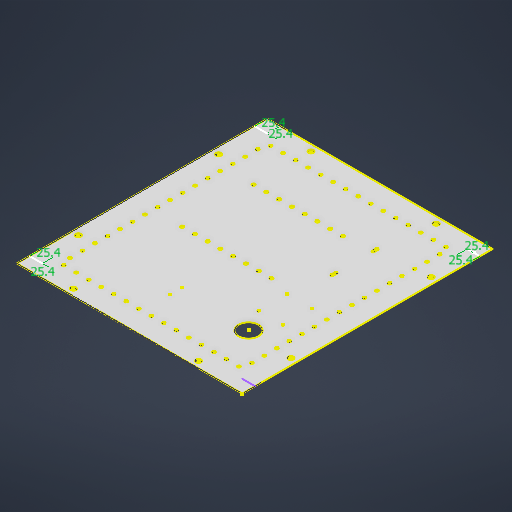
# Autodesk Inventor part: placa_dany
Saved by Autodesk Inventor 2026 (Build 300175050, 175E)
## iProperties
Created: 2025-11-18
Part Number: placa_dany
Material: Genérico
Document SubType Name: Modeling
Designer: sebas
Density: 1 g/cm^3
Appearance: Valor por defecto
Author: sebas
Autodesk Inventor part; units mm, degrees
ref_plane "YZ Plane" through (0, 0, 0) normal (1, 0, 0) x (0, 1, 0)
ref_plane "XZ Plane" through (0, 0, 0) normal (0, 1, 0) x (-1, 0, 0)
ref_plane "XY Plane" through (0, 0, 0) normal (0, 0, 1) x (1, 0, 0)
sketch "Boceto1" plane through (0, 0, 0) normal (0, 1, 0) x (-1, 0, 0)
  line L0 (0, 0) -> (450, 0)
  line L1 (450, 0) -> (450, -500)
  line L2 (450, -500) -> (0, -500)
  line L3 (0, -500) -> (0, 0)
  dimension "d0" = 450
  dimension "d1" = 500
  constraints: 8 end point, 2 parallel, 1 horizontal, 1 perpendicular
  measures "d0" distance of L1.end L2.end
  measures "d1" distance of L0.end L1.end
extrude "Extrusión1" add sketch "Boceto1" along normal blind 1.8
sketch "Boceto2" plane through (0, 1.8, 0) normal (0, 1, 0) x (1, 0, 0)
  line L0 (-450, 500) -> (-450, 0) projected
  line L1 (-450, 0) -> (0, 0) projected
  line L2 (-450, 0) -> (-450, 359)
  line L3 (0, 500) -> (-450, 500) projected
  line L4 (0, 0) -> (0, 500) projected
  line L5 (-348.5135, 228.3629) -> (-148.5135, 228.3629) construction
  circle A0 centre (-348.5135, 228.3629) radius 3
  circle A1 centre (-323.0135, 228.3629) radius 3
  circle A2 centre (-297.5135, 228.3629) radius 3
  circle A3 centre (-272.0135, 228.3629) radius 3
  circle A4 centre (-246.5135, 228.3629) radius 3
  circle A5 centre (-221.0135, 228.3629) radius 3
  circle A6 centre (-195.5135, 228.3629) radius 3
  circle A7 centre (-170.0135, 228.3629) radius 3
  line L6 (-345.4268, 372.6129) -> (-145.4268, 372.6129) construction
  circle A8 centre (-350, 372.6129) radius 3
  circle A9 centre (-324.5, 372.6129) radius 3
  circle A10 centre (-299, 372.6129) radius 3
  circle A11 centre (-273.5, 372.6129) radius 3
  circle A12 centre (-248, 372.6129) radius 3
  circle A13 centre (-222.5, 372.6129) radius 3
  circle A14 centre (-197, 372.6129) radius 3
  circle A15 centre (-171.5, 372.6129) radius 3
  line L7 (-400, 43.4) -> (-43, 43.4) construction
  circle A16 centre (-400, 43.4) radius 2.75
  circle A17 centre (-375, 43.4) radius 2.75
  circle A18 centre (-350, 43.4) radius 2.75
  circle A19 centre (-325, 43.4) radius 2.75
  circle A20 centre (-300, 43.4) radius 2.75
  circle A21 centre (-275, 43.4) radius 2.75
  circle A22 centre (-250, 43.4) radius 2.75
  circle A23 centre (-225, 43.4) radius 2.75
  circle A24 centre (-200, 43.4) radius 2.75
  circle A25 centre (-175, 43.4) radius 2.75
  circle A26 centre (-150, 43.4) radius 2.75
  circle A27 centre (-125, 43.4) radius 2.75
  circle A28 centre (-100, 43.4) radius 2.75
  circle A29 centre (-75, 43.4) radius 2.75
  circle A30 centre (-50, 43.4) radius 2.75
  line L8 (-406.6, 44.1958) -> (-406.6, 451.7958) construction
  circle A31 centre (-406.6, 62.5) radius 2.75
  circle A32 centre (-406.6, 87.5) radius 2.75
  circle A33 centre (-406.6, 112.5) radius 2.75
  circle A34 centre (-406.6, 137.5) radius 2.75
  circle A35 centre (-406.6, 162.5) radius 2.75
  circle A36 centre (-406.6, 187.5) radius 2.75
  circle A37 centre (-406.6, 212.5) radius 2.75
  circle A38 centre (-406.6, 237.5) radius 2.75
  circle A39 centre (-406.6, 262.5) radius 2.75
  circle A40 centre (-406.6, 287.5) radius 2.75
  circle A41 centre (-406.6, 312.5) radius 2.75
  circle A42 centre (-406.6, 337.5) radius 2.75
  circle A43 centre (-406.6, 362.5) radius 2.75
  circle A44 centre (-406.6, 387.5) radius 2.75
  circle A45 centre (-406.6, 412.5) radius 2.75
  circle A46 centre (-406.6, 437.5) radius 2.75
  line L9 (-406.6, 456.6) -> (-38, 456.6) construction
  circle A47 centre (-43.4, 62.5) radius 2.75
  circle A48 centre (-43.4, 87.5) radius 2.75
  circle A49 centre (-43.4, 112.5) radius 2.75
  circle A50 centre (-43.4, 137.5) radius 2.75
  circle A51 centre (-43.4, 162.5) radius 2.75
  circle A52 centre (-43.4, 187.5) radius 2.75
  circle A53 centre (-43.4, 212.5) radius 2.75
  circle A54 centre (-43.4, 237.5) radius 2.75
  circle A55 centre (-43.4, 262.5) radius 2.75
  circle A56 centre (-43.4, 287.5) radius 2.75
  circle A57 centre (-43.4, 312.5) radius 2.75
  circle A58 centre (-43.4, 337.5) radius 2.75
  circle A59 centre (-43.4, 362.5) radius 2.75
  circle A60 centre (-43.4, 387.5) radius 2.75
  circle A61 centre (-43.4, 412.5) radius 2.75
  circle A62 centre (-43.4, 437.5) radius 2.75
  line L10 (-400, 456.6) -> (-43, 456.6) construction
  circle A63 centre (-400, 456.6) radius 2.75
  circle A64 centre (-375, 456.6) radius 2.75
  circle A65 centre (-350, 456.6) radius 2.75
  circle A66 centre (-325, 456.6) radius 2.75
  circle A67 centre (-300, 456.6) radius 2.75
  circle A68 centre (-275, 456.6) radius 2.75
  circle A69 centre (-250, 456.6) radius 2.75
  circle A70 centre (-225, 456.6) radius 2.75
  circle A71 centre (-200, 456.6) radius 2.75
  circle A72 centre (-175, 456.6) radius 2.75
  circle A73 centre (-150, 456.6) radius 2.75
  circle A74 centre (-125, 456.6) radius 2.75
  circle A75 centre (-100, 456.6) radius 2.75
  circle A76 centre (-75, 456.6) radius 2.75
  circle A77 centre (-50, 456.6) radius 2.75
  arc A78 (-112.7335, 384.14) -> (-117.1835, 384.14) centre (-114.9585, 384.14) ccw
  arc A79 (-117.1835, 294.14) -> (-112.7335, 294.14) centre (-114.9585, 294.14) ccw
  arc A80 (-117.1835, 376.14) -> (-112.7335, 376.14) centre (-114.9585, 376.14) ccw
  arc A81 (-112.7335, 302.14) -> (-117.1835, 302.14) centre (-114.9585, 302.14) ccw
  line L11 (-117.1835, 384.14) -> (-117.1835, 376.14)
  line L12 (-112.7335, 376.14) -> (-112.7335, 384.14)
  line L13 (-117.1835, 302.14) -> (-117.1835, 294.14)
  line L14 (-112.7335, 294.14) -> (-112.7335, 302.14)
  circle A82 centre (-126.3146, 216.4498) radius 1.5
  circle A83 centre (-77.1746, 216.4498) radius 1.5
  circle A84 centre (-126.3146, 158.7698) radius 1.5
  circle A85 centre (-77.1746, 158.7698) radius 1.5
  circle A86 centre (-243.1932, 122.0864) radius 1
  circle A87 centre (-243.1932, 99.0264) radius 1
  circle A88 centre (-102.75, 115.25) radius 20
  circle A89 centre (-350, 487.3) radius 5
  circle A90 centre (-100, 487.3) radius 5
  circle A91 centre (-350, 12.7) radius 5
  circle A92 centre (-100, 12.7) radius 5
  circle A93 centre (-437.3, 390) radius 5
  circle A94 centre (-437.3, 110) radius 5
  circle A95 centre (-12.7, 390) radius 5
  circle A96 centre (-12.7, 110) radius 5
  point P0 (-43.4, 451.7958)
  point P1 (-406.6, 455.8042)
  dimension "d16" = 25.5
  dimension "d30" = 25.5
  dimension "d41" = 5.5
  dimension "d44" = 25
  dimension "d50" = 5.5
  dimension "d54" = 25
  dimension "d65" = 144.25
  dimension "d85" = 4.45
  dimension "d89" = 4.45
  dimension "d92" = 4.45
  dimension "d93" = 90
  dimension "d94" = 4.45
  dimension "d95" = 8
  dimension "d96" = 8
  dimension "d97" = 3
  dimension "d98" = 3
  dimension "d99" = 49.14
  dimension "d100" = 3
  dimension "d101" = 57.68
  dimension "d102" = 3
  dimension "d103" = 2
  dimension "d104" = 2
  dimension "d105" = 23.06
  dimension "d106" = 40
  dimension "d113" = 10
  dimension "d114" = 10
  dimension "d115" = 10
  dimension "d116" = 10
  dimension "d117" = 10
  dimension "d118" = 10
  dimension "d119" = 10
  dimension "d120" = 10
  dimension "d121" = 12.7
  dimension "d122" = 12.7
  dimension "d123" = 12.7
  dimension "d124" = 12.7
  dimension "d125" = 12.7
  dimension "d126" = 12.7
  dimension "d127" = 12.7
  dimension "d128" = 12.7
  dimension "d129" = 110
  dimension "d130" = 110
  dimension "d131" = 110
  dimension "d132" = 110
  dimension "d133" = 100
  dimension "d134" = 100
  dimension "d135" = 100
  dimension "d136" = 100
  constraints: 97 centre point, 22 end point, 8 point on circle, 7 horizontal, 6 point on line, 4 tangent, 3 coincident, 3 vertical, 1 perpendicular, 86 other
  measures "d16" distance of A0.centre A1.centre
  measures "d30" distance of A8.centre A9.centre
  measures "d41" diameter of A16
  measures "d44" distance of A16.centre A17.centre
  measures "d50" diameter of A31
  measures "d54" distance of A31.centre A32.centre
  measures "d65" distance between parallel lines of L6 L5
  measures "d85" diameter of A78
  measures "d89" diameter of A79
  measures "d92" diameter of A80
  measures "d93" distance of A79.centre A78.centre
  measures "d94" diameter of A81
  measures "d95" distance of A78.centre A80.centre
  measures "d96" distance of A81.centre A79.centre
  measures "d97" diameter of A82
  measures "d98" diameter of A83
  measures "d99" distance of A83.centre A82.centre
  measures "d100" diameter of A84
  measures "d101" distance of A82.centre A84.centre
  measures "d102" diameter of A85
  measures "d103" diameter of A86
  measures "d104" diameter of A87
  measures "d105" distance of A87.centre A86.centre
  measures "d106" diameter of A88
  measures "d113" diameter of A89
  measures "d114" diameter of A90
  measures "d115" diameter of A91
  measures "d116" diameter of A92
  measures "d117" diameter of A93
  measures "d118" diameter of A94
  measures "d119" diameter of A95
  measures "d120" diameter of A96
  measures "d121" distance from line of L3 A89.centre
  measures "d122" distance from line of L3 A90.centre
  measures "d123" distance from line of L0 A94.centre
  measures "d124" distance from line of L0 A93.centre
  measures "d125" distance from line of L1 A92.centre
  measures "d126" distance from line of L1 A91.centre
  measures "d127" distance from line of L4 A96.centre
  measures "d128" distance from line of L4 A95.centre
  measures "d129" distance from line of L3 A93.centre
  measures "d130" distance from line of L3 A95.centre
  measures "d131" distance from line of A94.centre L1
  measures "d132" distance from line of L1 A96.centre
  measures "d133" distance from line of L2 A91.centre
  measures "d134" distance from line of L4 A92.centre
  measures "d135" distance from line of L4 A90.centre
  measures "d136" distance from line of L0 A89.centre
extrude "Extrusión2" cut sketch "Boceto2" against normal blind 25 contours A0 | A1 | A2 | A3 | A4 | A5 | A6 | A7 | A8 | A9 | A10 | A11 | A12 | A13 | A14 | A15 | A16 | A17 | A18 | A19 | A20 | A21 | A22 | A23 | A24 | A25 | A26 | A27 | A28 | A29 | A30 | A31 | A32 | A33 | A34 | A35 | A36 | A37 | A38 | A39 | A40 | A41 | A42 | A43 | A44 | A45 | A46 | A47 | A48 | A49 | A50 | A51 | A52 | A53 | A54 | A55 | A56 | A57 | A58 | A59 | A60 | A61 | A62 | A63 | A64 | A65 | A66 | A67 | A68 | A69 | A70 | A71 | A72 | A73 | A74 | A75 | A76 | A77 | L12 A80 L11 A78 | L13 A81 L14 A79 | A82 | A83 | A84 | A85 | A86 | A87 | A88 | A89 | A90 | A91 | A92 | A93 | A94 | A95 | A96
sketch "Sketch5" plane through (0, 1.8, 0) normal (0, 1, 0) x (1, 0, 0)
  circle A0 centre (-12.7, 110) radius 5 projected
  circle A1 centre (-350, 487.3) radius 5 projected
  circle A2 centre (-243.1932, 122.0864) radius 1 projected
  circle A3 centre (-77.1746, 216.4498) radius 1.5 projected
  circle A4 centre (-406.6, 412.5) radius 2.75 projected
  circle A5 centre (-43.4, 362.5) radius 2.75 projected
  circle A6 centre (-43.4, 262.5) radius 2.75 projected
  circle A7 centre (-43.4, 162.5) radius 2.75 projected
  circle A8 centre (-43.4, 62.5) radius 2.75 projected
  circle A9 centre (-125, 43.4) radius 2.75 projected
  circle A10 centre (-225, 43.4) radius 2.75 projected
  circle A11 centre (-325, 43.4) radius 2.75 projected
  circle A12 centre (-221.0135, 228.3629) radius 3 projected
  circle A13 centre (-323.0135, 228.3629) radius 3 projected
  circle A14 centre (-299, 372.6129) radius 3 projected
  circle A15 centre (-197, 372.6129) radius 3 projected
  circle A16 centre (-406.6, 62.5) radius 2.75 projected
  circle A17 centre (-406.6, 162.5) radius 2.75 projected
  circle A18 centre (-406.6, 262.5) radius 2.75 projected
  circle A19 centre (-43.4, 437.5) radius 2.75 projected
  circle A20 centre (-100, 456.6) radius 2.75 projected
  circle A21 centre (-200, 456.6) radius 2.75 projected
  circle A22 centre (-300, 456.6) radius 2.75 projected
  circle A23 centre (-400, 456.6) radius 2.75 projected
  circle A24 centre (-325, 456.6) radius 2.75 projected
  circle A25 centre (-225, 456.6) radius 2.75 projected
  circle A26 centre (-125, 456.6) radius 2.75 projected
  circle A27 centre (-43.4, 412.5) radius 2.75 projected
  circle A28 centre (-406.6, 287.5) radius 2.75 projected
  circle A29 centre (-406.6, 187.5) radius 2.75 projected
  circle A30 centre (-406.6, 87.5) radius 2.75 projected
  circle A31 centre (-171.5, 372.6129) radius 3 projected
  circle A32 centre (-273.5, 372.6129) radius 3 projected
  circle A33 centre (-348.5135, 228.3629) radius 3 projected
  circle A34 centre (-246.5135, 228.3629) radius 3 projected
  circle A35 centre (-350, 43.4) radius 2.75 projected
  circle A36 centre (-250, 43.4) radius 2.75 projected
  circle A37 centre (-150, 43.4) radius 2.75 projected
  circle A38 centre (-50, 43.4) radius 2.75 projected
  circle A39 centre (-43.4, 137.5) radius 2.75 projected
  circle A40 centre (-43.4, 237.5) radius 2.75 projected
  circle A41 centre (-43.4, 337.5) radius 2.75 projected
  circle A42 centre (-406.6, 387.5) radius 2.75 projected
  arc A43 (-112.7335, 302.14) -> (-117.1835, 302.14) centre (-114.9585, 302.14) ccw projected
  line L0 (-112.7335, 302.14) -> (-112.7335, 294.14) projected
  arc A44 (-117.1835, 294.14) -> (-112.7335, 294.14) centre (-114.9585, 294.14) ccw projected
  line L1 (-117.1835, 294.14) -> (-117.1835, 302.14) projected
  circle A45 centre (-126.3146, 158.7698) radius 1.5 projected
  circle A46 centre (-437.3, 110) radius 5 projected
  circle A47 centre (-12.7, 390) radius 5 projected
  circle A48 centre (-100, 12.7) radius 5 projected
  circle A49 centre (-437.3, 390) radius 5 projected
  circle A50 centre (-243.1932, 99.0264) radius 1 projected
  circle A51 centre (-126.3146, 216.4498) radius 1.5 projected
  circle A52 centre (-406.6, 437.5) radius 2.75 projected
  circle A53 centre (-406.6, 337.5) radius 2.75 projected
  circle A54 centre (-43.4, 287.5) radius 2.75 projected
  circle A55 centre (-43.4, 187.5) radius 2.75 projected
  circle A56 centre (-43.4, 87.5) radius 2.75 projected
  circle A57 centre (-100, 43.4) radius 2.75 projected
  circle A58 centre (-200, 43.4) radius 2.75 projected
  circle A59 centre (-300, 43.4) radius 2.75 projected
  circle A60 centre (-195.5135, 228.3629) radius 3 projected
  circle A61 centre (-297.5135, 228.3629) radius 3 projected
  circle A62 centre (-324.5, 372.6129) radius 3 projected
  circle A63 centre (-222.5, 372.6129) radius 3 projected
  circle A64 centre (-375, 43.4) radius 2.75 projected
  circle A65 centre (-406.6, 137.5) radius 2.75 projected
  circle A66 centre (-406.6, 237.5) radius 2.75 projected
  circle A67 centre (-50, 456.6) radius 2.75 projected
  circle A68 centre (-75, 456.6) radius 2.75 projected
  circle A69 centre (-175, 456.6) radius 2.75 projected
  circle A70 centre (-275, 456.6) radius 2.75 projected
  circle A71 centre (-375, 456.6) radius 2.75 projected
  circle A72 centre (-350, 456.6) radius 2.75 projected
  circle A73 centre (-250, 456.6) radius 2.75 projected
  circle A74 centre (-150, 456.6) radius 2.75 projected
  circle A75 centre (-43.4, 387.5) radius 2.75 projected
  circle A76 centre (-406.6, 312.5) radius 2.75 projected
  circle A77 centre (-406.6, 212.5) radius 2.75 projected
  circle A78 centre (-406.6, 112.5) radius 2.75 projected
  circle A79 centre (-400, 43.4) radius 2.75 projected
  circle A80 centre (-248, 372.6129) radius 3 projected
  circle A81 centre (-350, 372.6129) radius 3 projected
  circle A82 centre (-272.0135, 228.3629) radius 3 projected
  circle A83 centre (-170.0135, 228.3629) radius 3 projected
  circle A84 centre (-275, 43.4) radius 2.75 projected
  circle A85 centre (-175, 43.4) radius 2.75 projected
  circle A86 centre (-75, 43.4) radius 2.75 projected
  circle A87 centre (-43.4, 112.5) radius 2.75 projected
  circle A88 centre (-43.4, 212.5) radius 2.75 projected
  circle A89 centre (-43.4, 312.5) radius 2.75 projected
  circle A90 centre (-406.6, 362.5) radius 2.75 projected
  arc A91 (-117.1835, 376.14) -> (-112.7335, 376.14) centre (-114.9585, 376.14) ccw projected
  line L2 (-117.1835, 376.14) -> (-117.1835, 384.14) projected
  arc A92 (-112.7335, 384.14) -> (-117.1835, 384.14) centre (-114.9585, 384.14) ccw projected
  line L3 (-112.7335, 384.14) -> (-112.7335, 376.14) projected
  circle A93 centre (-77.1746, 158.7698) radius 1.5 projected
  circle A94 centre (-102.75, 115.25) radius 20 projected
  circle A95 centre (-100, 487.3) radius 5 projected
  circle A96 centre (-350, 12.7) radius 5 projected
  line L4 (0, 500) -> (-450, 500) projected
  line L5 (-450, 500) -> (-450, 0) projected
  line L6 (-450, 0) -> (0, 0) projected
  line L7 (0, 0) -> (0, 500) projected
  line L8 (-450, 25.4) -> (-424.6, 25.4)
  line L9 (-450, 474.6) -> (-424.6, 474.6)
  line L10 (0, 474.6) -> (-25.4, 474.6)
  line L11 (0, 25.4) -> (-25.4, 25.4)
  point P0 (-12.7, 474.6)
  dimension "d137" = 25.4
  dimension "d138" = 25.4
  dimension "d139" = 25.4
  dimension "d140" = 25.4
  dimension "d141" = 25.4
  dimension "d142" = 25.4
  constraints: 8 end point, 4 point on line, 3 horizontal, 1 midpoint, 1 perpendicular
  measures "d137" distance of L8.start L8.end
  measures "d138" distance between parallel lines of L6 L8
  measures "d139" distance of L9.start L9.end
  measures "d140" distance between parallel lines of L4 L9
  measures "d141" distance of L10.start L10.end
  measures "d142" distance from line of L4 point (-12.7, 474.6)
